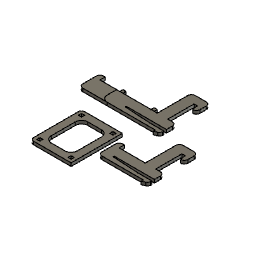
SKADIS_snap_in_hook_v4 (Autodesk Fusion 360 design; units mm, degrees)
Autodesk Fusion 360 part; units mm, degrees
note: some values were not read from the file. Set by a fixed rule: which sketch regions a step uses.
pattern_linear "R-Pattern1" [no effect]
pattern_linear "R-Pattern3" [no effect]
pattern_linear "R-Pattern4" [no effect]
pattern_linear "R-Pattern5" [no effect]
sketch "55mm hook" plane through (0, 0, 0) normal (0, 1, 0) x (1, 0, 0)
  line L0 (50.9989, 59.754) -> (50.9989, 54.008)
  line L1 (12.8247, 53.0002) -> (37.9331, 51.508)
  line L2 (50.9989, 54.008) -> (50, 54.008)
  line L3 (38, 83.008) -> (47.0796, 83.008) construction
  line L4 (42.9989, 63.254) -> (47.4989, 63.254)
  line L5 (23.0666, 48.254) -> (53.1332, 48.254) construction
  line L6 (23, 103.508) -> (53, 103.508) construction
  arc A0 (47.0796, 83.008) -> (50.5796, 86.508) centre (47.0796, 86.508) ccw
  line L7 (45.9989, 48.254) -> (45.9989, 46.254)
  arc A1 (-27, 51.754) -> (-23.5, 48.254) centre (-23.5, 51.754) ccw
  line L8 (47.0795, 83.008) -> (47.0796, 83.008)
  arc A2 (-23.5, 68.254) -> (-27, 64.754) centre (-23.5, 64.754) ccw
  line L9 (47.0796, 96.008) -> (36.4989, 96.008)
  line L10 (45.9989, 109.508) -> (45.9989, 88.508) construction
  line L11 (32.9989, 96.008) -> (50.5796, 96.008) construction
  line L12 (50.9989, 51.508) -> (50.9989, 50.2851)
  line L13 (42.9989, 88.508) -> (45.9989, 88.508)
  line L14 (50.5796, 86.508) -> (50.5796, 85.508)
  line L15 (45.9989, 88.508) -> (47.0795, 83.008)
  line L16 (-22.0011, 63.254) -> (-22.0011, 68.254)
  line L17 (50.5796, 85.508) -> (50.5796, 92.508)
  arc A3 (12.8247, 54.008) -> (12.8247, 53.0002) centre (12.8547, 53.5041) ccw
  line L18 (50, 54.008) -> (12.8247, 54.008)
  line L19 (32.9989, 63.254) -> (-22.0011, 63.254)
  line L20 (23, 88.508) -> (53, 88.508) construction
  arc A4 (50.5796, 92.508) -> (47.0796, 96.008) centre (47.0796, 92.508) ccw
  line L21 (50.2957, 51.508) -> (37.9331, 51.508)
  line L22 (50.9989, 51.508) -> (50.2957, 51.508)
  arc A5 (36.4989, 96.008) -> (32.9989, 92.508) centre (36.4989, 92.508) ccw
  arc A6 (49.1131, 47.4997) -> (50.9989, 50.2851) centre (47.9989, 50.2851) ccw
  line L23 (42.9989, 88.508) -> (42.9989, 63.254)
  line L24 (42.9989, 109.508) -> (42.9989, 43.0101) construction
  arc A7 (50.9989, 59.754) -> (47.4989, 63.254) centre (47.4989, 59.754) ccw
  line L25 (32.9989, 92.508) -> (32.9989, 63.254)
  line L26 (45.9989, 83.008) -> (45.9989, 43.0101) construction
  line L27 (-27, 64.754) -> (-27, 51.754)
  line L28 (-22.0011, 68.254) -> (-23.5, 68.254)
  line L29 (45.9989, 48.254) -> (42.9989, 48.254)
  line L30 (17.9989, 63.254) -> (47.9989, 63.254) construction
  line L31 (45.9989, 46.254) -> (49.1131, 47.4997)
  line L32 (42.9989, 48.254) -> (23.0666, 48.254)
  line L33 (23.0666, 48.254) -> (-23.5, 48.254)
  point P0 (23, 103.508)
  dimension "d170" = 15
  dimension "d171" = 40.254
  dimension "d172" = 15
  dimension "d173" = 3
  dimension "d174" = 7.5
  dimension "d175" = 5.5
  dimension "d176" = 55
  dimension "d177" = 5
  dimension "d178" = 10
  dimension "d179" = 3.5
  dimension "d180" = 2
  dimension "d181" = 3.254
  dimension "d182" = 2.5
  dimension "d183" = 3
  dimension "d184" = 30.1442
  dimension "d185" = 4.9989
  dimension "d186" = 5
  constraint coincident P0 L6.start
  constraint parallel L20 L30
  constraint perpendicular L5 L24
  constraint perpendicular L5 L10
  constraint perpendicular L3 L10
  constraint perpendicular L11 L24
  constraint coincident L13.start L20
  constraint coincident L13.start L24
  constraint coincident L10.end L20
  constraint coincident L26.start L10
  constraint coincident L26.start L3
  constraint perpendicular L11 L17
  constraint midpoint L19.start L30
  constraint perpendicular L25 L30
  constraint coincident L4.start L24
  constraint coincident L4.start L30
  constraint perpendicular L4 L23
  constraint perpendicular L0 L5
  constraint coincident L29.end L5
  constraint coincident L29.end L24
  constraint coincident L7.start L10
  constraint coincident L7.start L5
  constraint coincident L7.end L10
  constraint perpendicular L5 L7
  constraint coincident L12.start L0
  constraint perpendicular L0 L22
  constraint perpendicular L0 L2
  constraint perpendicular L19 L25
  constraint perpendicular L16 L19
  constraint perpendicular L16 L28
  constraint collinear L10 L26
  constraint collinear L0 L12
  constraint coincident L11.start L9
  constraint coincident L11.start L25
  constraint tangent L9 A5
  constraint tangent A5 L25
  constraint coincident L11.end L9
  constraint coincident L11.end L17
  constraint tangent L9 A4
  constraint tangent L17 A4
  constraint equal A4 A5
  constraint tangent A0 L14
  constraint tangent L3 A0
  constraint equal A0 A5
  constraint tangent L0 A7
  constraint tangent L4 A7
  constraint equal A5 A7
  constraint equal A1 A5
  constraint tangent A2 L28
  constraint equal A2 A5
  constraint tangent A1 L27
  constraint tangent A6 L31
  constraint tangent L12 A6
  constraint coincident L8.start L3
  constraint tangent L1 A3
  constraint tangent A1 L33
  constraint collinear L32 L33
  measures "d170" distance of L6 L20
  measures "d171" distance of L6 L30
  measures "d172" distance of L5 L30
  measures "d173" distance of L10 L24
  measures "d174" distance of L6 L11
  measures "d175" distance of L3 L20
  measures "d176" distance of L19.start L16.start
  measures "d177" distance of L0 L10
  measures "d178" distance of L24 L25
  measures "d179" radius of A5
  measures "d180" distance of L7.end L29
  measures "d181" distance of L5 L21
  measures "d182" distance of L18 L21
  measures "d183" radius of A6
  measures "d184" distance of A3.centre L24
  measures "d185" distance of L16 L27
  measures "d186" distance of L16.end L16.start
sketch "25mm hook" plane through (0, 0, 0) normal (0, 1, 0) x (1, 0, 0)
  line L0 (81.6176, 1.0886) -> (81.6176, -0.9114)
  line L1 (68.6176, 48.8426) -> (86.1982, 48.8426) construction
  line L2 (58.6853, 1.0886) -> (88.7519, 1.0886) construction
  line L3 (81.6176, 41.3426) -> (82.6981, 35.8426)
  arc A0 (42.1187, 21.0886) -> (38.6187, 17.5886) centre (42.1187, 17.5886) ccw
  arc A1 (86.1982, 45.3426) -> (82.6982, 48.8426) centre (82.6982, 45.3426) ccw
  line L4 (58.6187, 41.3426) -> (88.6187, 41.3426) construction
  line L5 (86.6176, 4.3426) -> (85.9144, 4.3426)
  line L6 (86.1982, 38.3426) -> (86.1982, 45.3426)
  line L7 (78.6176, 41.3426) -> (81.6176, 41.3426)
  line L8 (68.6176, 16.0886) -> (43.6176, 16.0886)
  line L9 (85.6187, 6.8426) -> (48.4434, 6.8426)
  line L10 (68.6176, 45.3426) -> (68.6176, 16.0886)
  line L11 (86.6176, 12.5886) -> (86.6176, 6.8426)
  arc A2 (48.4434, 6.8426) -> (48.4434, 5.8348) centre (48.4734, 6.3387) ccw
  line L12 (53.6176, 16.0886) -> (83.6176, 16.0886) construction
  line L13 (81.6176, 1.0886) -> (78.6176, 1.0886)
  line L14 (38.6187, 17.5886) -> (38.6187, 4.5886)
  arc A3 (38.6187, 4.5886) -> (42.1187, 1.0886) centre (42.1187, 4.5886) ccw
  line L15 (81.6176, -0.9114) -> (84.7318, 0.3343)
  line L16 (43.6176, 16.0886) -> (43.6176, 21.0886)
  line L17 (78.6176, 41.3426) -> (78.6176, 16.0886)
  line L18 (86.6176, 4.3426) -> (86.6176, 3.1197)
  line L19 (78.6176, 62.3426) -> (78.6176, -4.1553) construction
  line L20 (81.6176, 35.8426) -> (81.6176, -4.1553) construction
  line L21 (48.4434, 5.8348) -> (73.5517, 4.3426)
  line L22 (85.9144, 4.3426) -> (73.5517, 4.3426)
  line L23 (86.6176, 6.8426) -> (85.6187, 6.8426)
  arc A4 (86.6176, 12.5886) -> (83.1176, 16.0886) centre (83.1176, 12.5886) ccw
  arc A5 (84.7318, 0.3343) -> (86.6176, 3.1197) centre (83.6176, 3.1197) ccw
  line L24 (78.6176, 1.0886) -> (58.6853, 1.0886)
  line L25 (86.1982, 39.3426) -> (86.1982, 38.3426)
  line L26 (81.6176, 62.3426) -> (81.6176, 41.3426) construction
  line L27 (43.6176, 21.0886) -> (42.1187, 21.0886)
  line L28 (82.6982, 48.8426) -> (72.1176, 48.8426)
  arc A6 (82.6982, 35.8426) -> (86.1982, 39.3426) centre (82.6982, 39.3426) ccw
  line L29 (58.6853, 1.0886) -> (42.1187, 1.0886)
  line L30 (78.6176, 16.0886) -> (83.1176, 16.0886)
  line L31 (82.6981, 35.8426) -> (82.6982, 35.8426)
  arc A7 (72.1176, 48.8426) -> (68.6176, 45.3426) centre (72.1176, 45.3426) ccw
  line L32 (58.6187, 56.3426) -> (88.6187, 56.3426) construction
  line L33 (73.6187, 35.8426) -> (82.6982, 35.8426) construction
  point P0 (58.6187, 56.3426)
  dimension "d187" = 15
  dimension "d188" = 40.254
  dimension "d189" = 15
  dimension "d190" = 3
  dimension "d191" = 7.5
  dimension "d192" = 5.5
  dimension "d193" = 25
  dimension "d194" = 5
  dimension "d195" = 10
  dimension "d196" = 3.5
  dimension "d197" = 2
  dimension "d198" = 3.254
  dimension "d199" = 2.5
  dimension "d200" = 3
  dimension "d201" = 30.1442
  dimension "d202" = 4.9989
  dimension "d203" = 5
  constraint coincident P0 L32.start
  constraint parallel L4 L12
  constraint perpendicular L2 L19
  constraint perpendicular L2 L26
  constraint perpendicular L26 L33
  constraint perpendicular L1 L19
  constraint coincident L7.start L4
  constraint coincident L7.start L19
  constraint coincident L3.start L4
  constraint coincident L20.start L26
  constraint coincident L20.start L33
  constraint perpendicular L1 L6
  constraint midpoint L8.start L12
  constraint perpendicular L10 L12
  constraint coincident L17.end L19
  constraint coincident L17.end L12
  constraint perpendicular L17 L30
  constraint perpendicular L2 L11
  constraint coincident L13.end L2
  constraint coincident L13.end L19
  constraint coincident L0.start L26
  constraint coincident L0.start L2
  constraint coincident L0.end L26
  constraint perpendicular L0 L2
  constraint coincident L5.start L11
  constraint perpendicular L5 L11
  constraint perpendicular L11 L23
  constraint perpendicular L8 L10
  constraint perpendicular L8 L16
  constraint perpendicular L16 L27
  constraint collinear L20 L26
  constraint collinear L11 L18
  constraint coincident L1.start L28
  constraint coincident L1.start L10
  constraint tangent L28 A7
  constraint tangent L10 A7
  constraint coincident L1.end L28
  constraint coincident L1.end L6
  constraint tangent A1 L28
  constraint tangent A1 L6
  constraint equal A1 A7
  constraint tangent L25 A6
  constraint tangent A6 L33
  constraint equal A6 A7
  constraint tangent L11 A4
  constraint tangent A4 L30
  constraint equal A4 A7
  constraint equal A3 A7
  constraint tangent A0 L27
  constraint equal A0 A7
  constraint tangent L14 A3
  constraint tangent L15 A5
  constraint tangent L18 A5
  constraint coincident L3.end L33
  constraint tangent A2 L21
  constraint tangent A3 L29
  constraint collinear L24 L29
  measures "d187" distance of L4 L32
  measures "d188" distance of L12 L32
  measures "d189" distance of L2 L12
  measures "d190" distance of L19 L26
  measures "d191" distance of L1 L32
  measures "d192" distance of L4 L33
  measures "d193" distance of L8.start L8.end
  measures "d194" distance of L11 L26
  measures "d195" distance of L10 L19
  measures "d196" radius of A7
  measures "d197" distance of L0.end L13
  measures "d198" distance of L2 L22
  measures "d199" distance of L9 L22
  measures "d200" radius of A5
  measures "d201" distance of A2.centre L19
  measures "d202" distance of L14 L16
  measures "d203" distance of L8.end L16.end
extrude "Extrude7" add sketch "55mm hook" along normal blind 3 makes body 1
extrude "Extrude8" add sketch "25mm hook" along normal blind 3 separate body makes body 2
sketch "55mm hook clean" plane through (0, 0, 0) normal (0, 1, 0) x (1, 0, 0)
  line L0 (45.9989, 46.254) -> (49.1131, 47.4997)
  arc A0 (49.1131, 47.4997) -> (50.9989, 50.2851) centre (47.9989, 50.2851) ccw
  line L1 (50.9989, 50.2851) -> (50.9989, 51.508)
  line L2 (50.9989, 51.508) -> (37.9331, 51.508)
  line L3 (37.9331, 51.508) -> (12.8247, 53.0002)
  arc A1 (12.8247, 54.008) -> (12.8247, 53.0002) centre (12.8547, 53.5041) ccw
  line L4 (12.8247, 54.008) -> (50.9989, 54.008)
  line L5 (50.9989, 54.008) -> (50.9989, 59.754)
  arc A2 (50.9989, 59.754) -> (47.4989, 63.254) centre (47.4989, 59.754) ccw
  line L6 (47.4989, 63.254) -> (42.9989, 63.254)
  line L7 (42.9989, 63.254) -> (42.9989, 88.508)
  line L8 (42.9989, 88.508) -> (45.9989, 88.508)
  line L9 (45.9989, 88.508) -> (47.0795, 83.008)
  line L10 (47.0795, 83.008) -> (47.0796, 83.008)
  arc A3 (47.0796, 83.008) -> (50.5796, 86.508) centre (47.0796, 86.508) ccw
  line L11 (50.5796, 86.508) -> (50.5796, 92.508)
  arc A4 (50.5796, 92.508) -> (47.0796, 96.008) centre (47.0796, 92.508) ccw
  line L12 (47.0796, 96.008) -> (36.4989, 96.008)
  arc A5 (36.4989, 96.008) -> (32.9989, 92.508) centre (36.4989, 92.508) ccw
  line L13 (32.9989, 92.508) -> (32.9989, 63.254)
  line L14 (32.9989, 63.254) -> (-22.0011, 63.254)
  line L15 (-22.0011, 63.254) -> (-22.0011, 68.254)
  line L16 (-22.0011, 68.254) -> (-23.5, 68.254)
  arc A6 (-23.5, 68.254) -> (-27, 64.754) centre (-23.5, 64.754) ccw
  line L17 (-27, 64.754) -> (-27, 51.754)
  arc A7 (-27, 51.754) -> (-23.5, 48.254) centre (-23.5, 51.754) ccw
  line L18 (-23.5, 48.254) -> (45.9989, 48.254)
  line L19 (45.9989, 48.254) -> (45.9989, 46.254)
sketch "25mm_hook_clean" plane through (0, 0, 0) normal (0, 1, 0) x (1, 0, 0)
  line L0 (78.6176, 41.3426) -> (81.6176, 41.3426)
  line L1 (81.6176, 41.3426) -> (82.6981, 35.8426)
  line L2 (82.6981, 35.8426) -> (82.6982, 35.8426)
  arc A0 (82.6982, 35.8426) -> (86.1982, 39.3426) centre (82.6982, 39.3426) ccw
  line L3 (86.1982, 39.3426) -> (86.1982, 45.3426)
  arc A1 (86.1982, 45.3426) -> (82.6982, 48.8426) centre (82.6982, 45.3426) ccw
  line L4 (82.6982, 48.8426) -> (72.1176, 48.8426)
  arc A2 (72.1176, 48.8426) -> (68.6176, 45.3426) centre (72.1176, 45.3426) ccw
  line L5 (68.6176, 45.3426) -> (68.6176, 16.0886)
  line L6 (68.6176, 16.0886) -> (43.6176, 16.0886)
  line L7 (43.6176, 16.0886) -> (43.6176, 21.0886)
  line L8 (43.6176, 21.0886) -> (42.1187, 21.0886)
  arc A3 (42.1187, 21.0886) -> (38.6187, 17.5886) centre (42.1187, 17.5886) ccw
  line L9 (38.6187, 17.5886) -> (38.6187, 4.5886)
  arc A4 (38.6187, 4.5886) -> (42.1187, 1.0886) centre (42.1187, 4.5886) ccw
  line L10 (42.1187, 1.0886) -> (81.6176, 1.0886)
  line L11 (81.6176, 1.0886) -> (81.6176, -0.9114)
  line L12 (81.6176, -0.9114) -> (84.7318, 0.3343)
  arc A5 (84.7318, 0.3343) -> (86.6176, 3.1197) centre (83.6176, 3.1197) ccw
  line L13 (86.6176, 3.1197) -> (86.6176, 4.3426)
  line L14 (86.6176, 4.3426) -> (73.5517, 4.3426)
  line L15 (73.5517, 4.3426) -> (48.4434, 5.8348)
  arc A6 (48.4434, 6.8426) -> (48.4434, 5.8348) centre (48.4734, 6.3387) ccw
  line L16 (48.4434, 6.8426) -> (86.6176, 6.8426)
  line L17 (86.6176, 6.8426) -> (86.6176, 12.5886)
  arc A7 (86.6176, 12.5886) -> (83.1176, 16.0886) centre (83.1176, 12.5886) ccw
  line L18 (83.1176, 16.0886) -> (78.6176, 16.0886)
  line L19 (78.6176, 16.0886) -> (78.6176, 41.3426)
sketch "scissor holder" plane through (0, 0, 0) normal (0, 1, 0) x (1, 0, 0)
  line L0 (50.9989, 54.008) -> (50, 54.008)
  line L1 (50.5796, 86.508) -> (50.5796, 85.508)
  arc A0 (36.4989, 96.008) -> (32.9989, 92.508) centre (36.4989, 92.508) ccw
  line L2 (45.9989, 88.508) -> (47.0795, 83.008)
  line L3 (50.2957, 51.508) -> (37.9331, 51.508)
  line L4 (38, 83.008) -> (47.0796, 83.008) construction
  line L5 (32.9989, 96.008) -> (50.5796, 96.008) construction
  line L6 (23.0666, 48.254) -> (-0.0011, 48.254)
  line L7 (50.9989, 51.508) -> (50.9989, 50.2851)
  line L8 (45.9989, 48.254) -> (45.9989, 46.254)
  line L9 (42.9989, 109.508) -> (42.9989, 43.0101) construction
  line L10 (23, 88.508) -> (53, 88.508) construction
  line L11 (42.9989, 88.508) -> (45.9989, 88.508)
  line L12 (42.9989, 48.254) -> (23.0666, 48.254)
  line L13 (23, 103.508) -> (53, 103.508) construction
  line L14 (17.9989, 63.254) -> (47.9989, 63.254) construction
  line L15 (50.9989, 59.754) -> (50.9989, 54.008)
  arc A1 (50.5796, 92.508) -> (47.0796, 96.008) centre (47.0796, 92.508) ccw
  arc A2 (49.1131, 47.4997) -> (50.9989, 50.2851) centre (47.9989, 50.2851) ccw
  line L16 (32.9989, 92.508) -> (32.9989, 63.254)
  arc A3 (12.8247, 54.008) -> (12.8247, 53.0002) centre (12.8547, 53.5041) ccw
  line L17 (50.5796, 85.508) -> (50.5796, 92.508)
  arc A4 (50.9989, 59.754) -> (47.4989, 63.254) centre (47.4989, 59.754) ccw
  line L18 (45.9989, 46.254) -> (49.1131, 47.4997)
  line L19 (45.9989, 48.254) -> (42.9989, 48.254)
  line L20 (50, 54.008) -> (12.8247, 54.008)
  line L21 (45.9989, 109.508) -> (45.9989, 88.508) construction
  line L22 (12.8247, 53.0002) -> (37.9331, 51.508)
  line L23 (42.9989, 88.508) -> (42.9989, 63.254)
  line L24 (23.0666, 48.254) -> (53.1332, 48.254) construction
  line L25 (47.0795, 83.008) -> (47.0796, 83.008)
  line L26 (47.0796, 96.008) -> (36.4989, 96.008)
  line L27 (42.9989, 63.254) -> (47.4989, 63.254)
  arc A5 (47.0796, 83.008) -> (50.5796, 86.508) centre (47.0796, 86.508) ccw
  line L28 (45.9989, 83.008) -> (45.9989, 43.0101) construction
  line L29 (50.9989, 51.508) -> (50.2957, 51.508)
  line L30 (32.9989, 29.657) -> (-3.0011, 29.657)
  line L31 (-6.0011, 26.657) -> (-6.0011, -16.343)
  line L32 (-3.0011, -19.343) -> (32.9989, -19.343)
  line L33 (32.9989, -19.343) -> (32.9989, 29.657)
  line L34 (-6.0011, 26.657) -> (-30.4362, 26.657) construction
  line L35 (-30.4362, 26.657) -> (32.9989, 26.657) construction
  line L36 (-6.0011, 23.657) -> (32.9989, 23.657) construction
  line L37 (-6.0011, -13.343) -> (32.9989, -13.343) construction
  line L38 (-6.0011, -16.343) -> (32.9989, -16.343) construction
  line L39 (32.9989, 5.157) -> (32.1695, 5.157) construction
  line L40 (32.1695, 5.157) -> (-6.0011, 5.157) construction
  line L41 (6.9989, 22.657) -> (19.9989, 22.657)
  line L42 (25.9989, 16.657) -> (25.9989, -6.343)
  line L43 (19.9989, -12.343) -> (6.9989, -12.343)
  line L44 (0.9989, -6.343) -> (0.9989, 16.657)
  line L45 (0.9989, 22.657) -> (25.9989, -12.343) construction
  line L46 (25.9989, 22.657) -> (0.9989, -12.343) construction
  line L47 (32.9989, 63.254) -> (32.9989, 29.657) construction
  line L48 (-6.0011, 29.657) -> (-6.0011, 68.1392) construction
  line L49 (-3.0011, 23.657) -> (-3.0011, 67.8455) construction
  line L50 (-0.0011, 23.657) -> (-0.0011, 69.3142) construction
  line L51 (29.9989, 23.657) -> (29.9989, 72.6924) construction
  line L52 (26.9989, 23.657) -> (26.9989, 72.2518) construction
  line L53 (29.9989, 23.657) -> (29.9989, -19.343) construction
  line L54 (26.9989, 23.657) -> (26.9989, -19.343) construction
  line L55 (-0.0011, 23.657) -> (-0.0011, -19.343) construction
  line L56 (-3.0011, 23.657) -> (-3.0011, -19.343) construction
  line L57 (29.9989, 66.254) -> (-6.0011, 66.254) construction
  line L58 (-6.0011, 54.254) -> (-6.0011, 63.254)
  line L59 (-3.0011, 63.254) -> (-3.0011, 66.254)
  line L60 (-3.0011, 66.254) -> (-0.0011, 66.254)
  line L61 (-0.0011, 66.254) -> (-0.0011, 63.254)
  line L62 (26.9989, 63.254) -> (26.9989, 66.254)
  line L63 (26.9989, 66.254) -> (29.9989, 66.254)
  line L64 (29.9989, 66.254) -> (29.9968, 63.254)
  line L65 (-3.0011, 63.254) -> (-6.0011, 63.254)
  line L66 (32.9989, 63.254) -> (29.9968, 63.254)
  line L67 (26.9989, 63.254) -> (-0.0011, 63.254)
  arc A6 (6.9989, 22.657) -> (0.9989, 16.657) centre (6.9989, 16.657) ccw
  arc A7 (25.9989, 16.657) -> (19.9989, 22.657) centre (19.9989, 16.657) ccw
  arc A8 (19.9989, -12.343) -> (25.9989, -6.343) centre (19.9989, -6.343) ccw
  arc A9 (0.9989, -6.343) -> (6.9989, -12.343) centre (6.9989, -6.343) ccw
  arc A10 (-6.0011, 54.254) -> (-0.0011, 48.254) centre (-0.0011, 54.254) ccw
  line L68 (-3.0011, 23.657) -> (-3.0011, 26.657)
  line L69 (-0.0011, 26.657) -> (-0.0011, 23.657)
  line L70 (-0.0011, 23.657) -> (-3.0011, 23.657)
  line L71 (-3.0011, 26.657) -> (-0.0011, 26.657)
  line L72 (26.9989, 26.657) -> (29.9989, 26.657)
  line L73 (29.9989, 26.657) -> (29.9989, 23.657)
  line L74 (26.9989, 23.657) -> (26.9989, 26.657)
  line L75 (26.9989, 23.657) -> (29.9989, 23.657)
  line L76 (-3.0011, -13.343) -> (-0.0011, -13.343)
  line L77 (-0.0011, -13.343) -> (-0.0011, -16.343)
  line L78 (-0.0011, -16.343) -> (-3.0011, -16.343)
  line L79 (-3.0011, -16.343) -> (-3.0011, -13.343)
  line L80 (26.9989, -16.343) -> (26.9989, -13.343)
  line L81 (26.9989, -13.343) -> (29.9989, -13.343)
  line L82 (29.9989, -16.343) -> (29.9989, -13.343)
  line L83 (29.9989, -16.343) -> (26.9989, -16.343)
  arc A11 (-3.0011, 29.657) -> (-6.0011, 26.657) centre (-3.0011, 26.657) ccw
  arc A12 (-6.0011, -16.343) -> (-3.0011, -19.343) centre (-3.0011, -16.343) ccw
  point P0 (23, 103.508)
  point P1 (13.4989, 5.157)
  dimension "d208" = 15
  dimension "d209" = 40.254
  dimension "d210" = 15
  dimension "d211" = 3
  dimension "d212" = 7.5
  dimension "d213" = 5.5
  dimension "d215" = 5
  dimension "d216" = 10
  dimension "d217" = 3.5
  dimension "d218" = 2
  dimension "d219" = 3.254
  dimension "d220" = 2.5
  dimension "d221" = 3
  dimension "d222" = 30.1442
  dimension "d227" = 3
  dimension "d228" = 3
  dimension "d229" = 3
  dimension "d230" = 3
  dimension "d231" = 40
  dimension "d232" = 25
  dimension "d233" = 35
  dimension "d234" = 7
  dimension "d235" = 3
  dimension "d236" = 3
  dimension "d237" = 3
  dimension "d238" = 3
  dimension "d239" = 7
  dimension "d240" = 3
  dimension "d241" = 6
  dimension "d244" = 3
  constraint coincident P0 L13.start
  constraint parallel L10 L14
  constraint perpendicular L9 L24
  constraint perpendicular L21 L24
  constraint perpendicular L4 L21
  constraint perpendicular L5 L9
  constraint coincident L11.start L10
  constraint coincident L11.start L9
  constraint coincident L2.start L10
  constraint coincident L28.start L21
  constraint coincident L28.start L4
  constraint perpendicular L5 L17
  constraint midpoint L16.end L14
  constraint perpendicular L14 L16
  constraint coincident L23.end L9
  constraint coincident L23.end L14
  constraint perpendicular L23 L27
  constraint perpendicular L15 L24
  constraint coincident L12.start L24
  constraint coincident L12.start L9
  constraint coincident L8.start L21
  constraint coincident L8.start L24
  constraint coincident L8.end L21
  constraint perpendicular L8 L24
  constraint coincident L7.start L15
  constraint perpendicular L15 L29
  constraint perpendicular L0 L15
  constraint perpendicular L16 L66
  constraint collinear L21 L28
  constraint collinear L7 L15
  constraint coincident L5.start L26
  constraint coincident L5.start L16
  constraint tangent A0 L26
  constraint tangent A0 L16
  constraint coincident L5.end L26
  constraint coincident L5.end L17
  constraint tangent A1 L26
  constraint tangent A1 L17
  constraint equal A0 A1
  constraint tangent L1 A5
  constraint tangent L4 A5
  constraint equal A0 A5
  constraint tangent L15 A4
  constraint tangent A4 L27
  constraint equal A0 A4
  constraint tangent A2 L18
  constraint tangent L7 A2
  constraint coincident L2.end L4
  constraint tangent A3 L22
  constraint collinear L6 L12
  constraint horizontal L30
  constraint vertical L31
  constraint horizontal L32
  constraint vertical L33
  constraint coincident L31 L34.start
  constraint perpendicular L31 L34
  constraint coincident L33 L35.end
  constraint perpendicular L33 L35
  constraint coincident L31 L36.start
  constraint coincident L33 L36.end
  constraint perpendicular L33 L36
  constraint coincident L31 L37.start
  constraint coincident L33 L37.end
  constraint perpendicular L33 L37
  constraint coincident L31 L38.start
  constraint coincident L33 L38.end
  constraint perpendicular L31 L38
  constraint midpoint L33 L39.start
  constraint perpendicular L33 L39
  constraint horizontal L41
  constraint perpendicular L41 L42
  constraint parallel L41 L43
  constraint parallel L42 L44
  constraint coincident L45 P1
  constraint coincident L46 P1
  constraint coincident L40 P1
  constraint perpendicular L30 L47
  constraint perpendicular L48 L66
  constraint coincident L36 L49.start
  constraint perpendicular L49 L66
  constraint coincident L36 L50.start
  constraint perpendicular L50 L66
  constraint coincident L36 L51.start
  constraint perpendicular L20 L51
  constraint coincident L36 L52.start
  constraint perpendicular L36 L52
  constraint coincident L32 L53.end
  constraint perpendicular L32 L53
  constraint perpendicular L38 L54
  constraint coincident L32 L55.end
  constraint perpendicular L32 L55
  constraint coincident L32 L56.end
  constraint perpendicular L32 L56
  constraint coincident L51 L57.start
  constraint coincident L48 L57.end
  constraint perpendicular L48 L57
  constraint coincident L48 L58.end
  constraint coincident L59.start L66
  constraint coincident L49 L59.start
  constraint coincident L49 L59.end
  constraint coincident L57 L59.end
  constraint coincident L57 L60.end
  constraint coincident L50 L60.end
  constraint coincident L50 L61.end
  constraint coincident L62.start L66
  constraint coincident L52 L62.start
  constraint coincident L52 L62.end
  constraint coincident L57 L62.end
  constraint coincident L14 L64.end
  constraint collinear L65 L66
  constraint collinear L66 L67
  constraint coincident L45.start L41
  constraint coincident L45.start L44
  constraint tangent L41 A6
  constraint tangent L44 A6
  constraint coincident L46.start L41
  constraint coincident L46.start L42
  constraint tangent L41 A7
  constraint tangent L42 A7
  constraint equal A6 A7
  constraint coincident L45.end L42
  constraint coincident L45.end L43
  constraint tangent L42 A8
  constraint tangent L43 A8
  constraint equal A6 A8
  constraint coincident L46.end L43
  constraint coincident L46.end L44
  constraint tangent L43 A9
  constraint tangent L44 A9
  constraint equal A6 A9
  constraint tangent L6 A10
  constraint tangent L58 A10
  constraint equal A6 A10
  constraint coincident L49 L68.end
  constraint coincident L35 L68.end
  constraint coincident L35 L69.start
  constraint coincident L50 L69.start
  constraint coincident L35 L72.start
  constraint coincident L52 L72.start
  constraint coincident L51 L72.end
  constraint coincident L35 L72.end
  constraint coincident L56 L76.start
  constraint coincident L37 L76.start
  constraint coincident L37 L76.end
  constraint coincident L55 L76.end
  constraint coincident L55 L77.end
  constraint coincident L38 L77.end
  constraint coincident L38 L78.end
  constraint coincident L56 L78.end
  constraint coincident L54 L80.start
  constraint coincident L38 L80.start
  constraint coincident L54 L80.end
  constraint coincident L37 L80.end
  constraint coincident L37 L81.end
  constraint coincident L53 L81.end
  constraint coincident L38 L82.start
  constraint coincident L53 L82.start
  constraint coincident L31 L40.end
  constraint coincident L48.start L30
  constraint coincident L48.start L31
  constraint tangent L30 A11
  constraint tangent L31 A11
  constraint tangent L31 A12
  constraint tangent L32 A12
  constraint equal A11 A12
  measures "d208" distance of L10 L13
  measures "d209" distance of L13 L14
  measures "d210" distance of L14 L24
  measures "d211" distance of L9 L21
  measures "d212" distance of L5 L13
  measures "d213" distance of L4 L10
  measures "d215" distance of L15 L21
  measures "d216" distance of L9 L16
  measures "d217" radius of A0
  measures "d218" distance of L8.end L19
  measures "d219" distance of L3 L24
  measures "d220" distance of L3 L20
  measures "d221" radius of A2
  measures "d222" distance of A3.centre L9
  measures "d227" distance of L30 L35
  measures "d228" distance of L35 L36
  measures "d229" distance of L37 L38
  measures "d230" distance of L32 L38
  measures "d231" distance of L36 L38
  measures "d232" distance of L45.end L46.end
  measures "d233" distance of L46.start L45.end
  measures "d234" distance of L31 L44
  measures "d235" distance of L47 L51
  measures "d236" distance of L51 L52
  measures "d237" distance of L48 L49
  measures "d238" distance of L49 L50
  measures "d239" distance of L33 L42
  measures "d240" distance of L57 L66
  measures "d241" radius of A6
  measures "d244" radius of A11
extrude "Extrude10" add sketch "scissor holder" along normal blind 3 separate body contours L30 L31 L32 L33 A11 A12 makes body 3
extrude "Extrude9" add sketch "scissor holder" along normal blind 3 separate body contours L0 A0 L2 L3 L6 L7 L8 L11 L12 L15 A1 A2 L16 A3 L17 A4 L18 L19 L20 L22 L23 L26 L27 A5 L29 L58 L59 L60 L61 L62 L63 L64 L65 L66 L67 A10 makes body 4
sketch "scissor plate clean" plane through (0, 0, 0) normal (0, 1, 0) x (1, 0, 0)
  line L0 (26.9989, 23.657) -> (26.9989, 26.657)
  line L1 (26.9989, 26.657) -> (29.9989, 26.657)
  line L2 (29.9989, 26.657) -> (29.9989, 23.657)
  line L3 (29.9989, 23.657) -> (26.9989, 23.657)
  arc A0 (6.9989, 22.657) -> (0.9989, 16.657) centre (6.9989, 16.657) ccw
  line L4 (6.9989, 22.657) -> (19.9989, 22.657)
  arc A1 (25.9989, 16.657) -> (19.9989, 22.657) centre (19.9989, 16.657) ccw
  line L5 (25.9989, 16.657) -> (25.9989, -6.343)
  arc A2 (19.9989, -12.343) -> (25.9989, -6.343) centre (19.9989, -6.343) ccw
  line L6 (19.9989, -12.343) -> (6.9989, -12.343)
  arc A3 (0.9989, -6.343) -> (6.9989, -12.343) centre (6.9989, -6.343) ccw
  line L7 (0.9989, -6.343) -> (0.9989, 16.657)
  line L8 (-0.0011, -16.343) -> (-3.0011, -16.343)
  line L9 (-3.0011, -16.343) -> (-3.0011, -13.343)
  line L10 (-3.0011, -13.343) -> (-0.0011, -13.343)
  line L11 (-0.0011, -13.343) -> (-0.0011, -16.343)
  line L12 (29.9989, -13.343) -> (29.9989, -16.343)
  line L13 (29.9989, -16.343) -> (26.9989, -16.343)
  line L14 (26.9989, -16.343) -> (26.9989, -13.343)
  line L15 (26.9989, -13.343) -> (29.9989, -13.343)
  line L16 (-3.0011, 23.657) -> (-3.0011, 26.657)
  line L17 (-3.0011, 26.657) -> (-0.0011, 26.657)
  line L18 (-0.0011, 26.657) -> (-0.0011, 23.657)
  line L19 (-0.0011, 23.657) -> (-3.0011, 23.657)
  arc A4 (-6.0011, -16.343) -> (-3.0011, -19.343) centre (-3.0011, -16.343) ccw
  line L20 (-3.0011, -19.343) -> (32.9989, -19.343)
  line L21 (32.9989, -19.343) -> (32.9989, 29.657)
  line L22 (32.9989, 29.657) -> (-3.0011, 29.657)
  arc A5 (-3.0011, 29.657) -> (-6.0011, 26.657) centre (-3.0011, 26.657) ccw
  line L23 (-6.0011, 26.657) -> (-6.0011, -16.343)
sketch "scissor bracket clean" plane through (0, 0, 0) normal (0, 1, 0) x (1, 0, 0)
  line L0 (-3.0011, 63.254) -> (-6.0011, 63.254)
  line L1 (-6.0011, 63.254) -> (-6.0011, 54.254)
  arc A0 (-6.0011, 54.254) -> (-0.0011, 48.254) centre (-0.0011, 54.254) ccw
  line L2 (-0.0011, 48.254) -> (45.9989, 48.254)
  line L3 (45.9989, 48.254) -> (45.9989, 46.254)
  line L4 (45.9989, 46.254) -> (49.1131, 47.4997)
  arc A1 (49.1131, 47.4997) -> (50.9989, 50.2851) centre (47.9989, 50.2851) ccw
  line L5 (50.9989, 50.2851) -> (50.9989, 51.508)
  line L6 (50.9989, 51.508) -> (37.9331, 51.508)
  line L7 (37.9331, 51.508) -> (12.8247, 53.0002)
  arc A2 (12.8247, 54.008) -> (12.8247, 53.0002) centre (12.8547, 53.5041) ccw
  line L8 (12.8247, 54.008) -> (50.9989, 54.008)
  line L9 (50.9989, 54.008) -> (50.9989, 59.754)
  arc A3 (50.9989, 59.754) -> (47.4989, 63.254) centre (47.4989, 59.754) ccw
  line L10 (47.4989, 63.254) -> (42.9989, 63.254)
  line L11 (42.9989, 63.254) -> (42.9989, 88.508)
  line L12 (42.9989, 88.508) -> (45.9989, 88.508)
  line L13 (45.9989, 88.508) -> (47.0795, 83.008)
  line L14 (47.0795, 83.008) -> (47.0796, 83.008)
  arc A4 (47.0796, 83.008) -> (50.5796, 86.508) centre (47.0796, 86.508) ccw
  line L15 (50.5796, 86.508) -> (50.5796, 92.508)
  arc A5 (50.5796, 92.508) -> (47.0796, 96.008) centre (47.0796, 92.508) ccw
  line L16 (47.0796, 96.008) -> (36.4989, 96.008)
  arc A6 (36.4989, 96.008) -> (32.9989, 92.508) centre (36.4989, 92.508) ccw
  line L17 (32.9989, 92.508) -> (32.9989, 63.254)
  line L18 (32.9989, 63.254) -> (29.9968, 63.254)
  line L19 (29.9968, 63.254) -> (29.9989, 66.254)
  line L20 (29.9989, 66.254) -> (26.9989, 66.254)
  line L21 (26.9989, 66.254) -> (26.9989, 63.254)
  line L22 (26.9989, 63.254) -> (-0.0011, 63.254)
  line L23 (-0.0011, 63.254) -> (-0.0011, 66.254)
  line L24 (-0.0011, 66.254) -> (-3.0011, 66.254)
  line L25 (-3.0011, 66.254) -> (-3.0011, 63.254)
equation "material_thinkness = 3.0 mm"
equation "board_height = ( 1 + num_rows ) * row_spacing"
equation "board_width = ( 1 + num_columns ) * col_spacing"
equation "fillet_distance = 10 mm"
equation "pill_height = 15 mm"
equation "pill_width = 5 mm"
equation "hole_spacing = 30 mm"
equation "board_padding = 14 mm"
equation "d28 = num_columns + 1"
equation "d30 = col_spacing"
equation "pill_count = 14"
equation "board_vertical_padding = 35.5 mm"
equation "board_vertical_padding_small = 11.5 mm"
equation "d47 = num_rows"
equation "d49 = row_spacing"
equation "vertica_pill_inner = 13"
equation "pill_spacing = 35 mm"
equation "d60 = num_columns"
equation "d62 = col_spacing"
equation "d64 = num_rows + 1"
equation "d66 = -row_spacing"
equation "spigot_width = material_thinkness"
equation "spigot_height = pill_height"
equation "spigot_drop = spigot_height / 2"
equation "spigot_spacing = 40.254 mm"
equation "spigot_latch = 2 mm"
equation "num_columns = 9"
equation "num_rows = 13"
equation "row_spacing = 40 mm"
equation "col_spacing = 40 mm"
equation "mounting_hole_dia = 6 mm"
equation "d170 = spigot_height"
equation "d171 = spigot_spacing"
equation "d172 = spigot_height"
equation "d173 = material_thinkness"
equation "d174 = spigot_drop"
equation "d175 = spigot_drop - 2 mm"
equation "d180 = spigot_latch"
equation "d182 = spigot_latch + 0.5 mm"
equation "d187 = spigot_height"
equation "d188 = spigot_spacing"
equation "d189 = spigot_height"
equation "d190 = material_thinkness"
equation "d191 = spigot_drop"
equation "d192 = spigot_drop - 2 mm"
equation "d197 = spigot_latch"
equation "d199 = spigot_latch + 0.5 mm"
equation "d204 = material_thinkness"
equation "d206 = material_thinkness"
equation "d208 = spigot_height"
equation "d209 = spigot_spacing"
equation "d210 = spigot_height"
equation "d211 = material_thinkness"
equation "d212 = spigot_drop"
equation "d213 = spigot_drop - 2 mm"
equation "d218 = spigot_latch"
equation "d220 = spigot_latch + 0.5 mm"
equation "d227 = material_thinkness"
equation "d228 = material_thinkness"
equation "d229 = material_thinkness"
equation "d230 = material_thinkness"
equation "d231 = col_spacing"
equation "d235 = material_thinkness"
equation "d236 = material_thinkness"
equation "d237 = material_thinkness"
equation "d238 = material_thinkness"
equation "d240 = material_thinkness"
equation "d242 = material_thinkness"
equation "d244 = material_thinkness"
equation "d245 = material_thinkness"
named bodies: "55mm hook", "25mm hook", "scissor bracket", "scissor plate"
